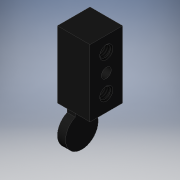
# Autodesk Inventor part: HGP-16---(116_JAW)
Saved by Autodesk Inventor 2019 (Build 230136000, 136)
## iProperties
Created: 2023-03-06
Part Number: HGP-16---(116_JAW)
Material: Generic
Catalog Web Link: www.cadenas.de
Description: HGP-(JAW)-parallel gripper
Vendor: FESTO
Document SubType Name: Modeling
Designer: psAdmin
Manufacturer: FESTO
Mass: 2.0446 g
Surface Area: 15.2758 cm^2
Volume: 2.0446 cm^3
Density: 1 g/cm^3
Appearance: PSOLRGB-128-128-128
Category: PARTsolutions
Company: FESTO
Title: HGP-16
Author: Cadenas PARTsolutions
Comments: parallel gripper
PSOL_IDENT_0: {$CADENAS_DATA/23d-libs/festo/parts/h/hgp/parts/hgp_jaw.prj},168 {VTYP=3D},{NB=HGP-16---(116_JAW)},{
PSOL_IDENT_1: LINA=HGP-16},{NN=HGP-(JAW)},{DATE=10.09.2021 08:18:21},{GEOMDATE=11.03.2020 13:19:07},{VERSION=},{LI
PSOL_IDENT_2: NEID=210},{WBVAR=},{WBNUMERIC=}  {NB=HGP-16---(116_JAW)},{LINA=HGP-16},{KT=3},{TNR=},{TYP=HGP-16},{K
PSOL_IDENT_3: DM=116},{B1=47.000},{B2=25.000},{B3=16.400},{B4=43.800},{B5=46.400},{B6=10.000},{B8=67.000},{D2=M 4}
PSOL_IDENT_4: ,{D4=M 4},{D5=3.300},{D6=3.000},{H1=83.000},{H2=20.500},{H7=11.000},{H8=5.500},{H9=10.000},{H11=38.1
PSOL_IDENT_5: 00},{L3=10.000},{L6S=30.000},{D4P=4.000},{KDR5=3.242},{VERS=3.000}
NB: HGP-16---(116_JAW)
NN: HGP-(JAW)
NT: parallel gripper
NBSYN: $TYP.---($KDM._JAW)
LINA: HGP-16
CATALOG: Festo
TYP: HGP-16
KDM: 116
B1: 47
B2: 25
B3: 16.4
B4: 43.8
B5: 46.4
B6: 10
B8: 67
D2: M 4
D4: M 4
D5: 3.3
D6: 3
H1: 83
H2: 20.5
H7: 11
H8: 5.5
H9: 10
H11: 38.1
L3: 10
L6S: 30
D4P: 4
SUPPLIER: FESTO
ARTICLENO: HGP-16---(116_JAW)
BOMINFO: HGP-16
CREATOR: CADENAS GmbH
Autodesk Inventor part; units mm, degrees
sketch "Sketch_11" plane through (0, 0, 0) normal (0, 0, 1) x (1, 0, 0)
  line L0 (0, 0) -> (10, 0)
  line L1 (10, 0) -> (10, 20.5)
  line L2 (10, 20.5) -> (0, 20.5)
  line L3 (0, 20.5) -> (0, 0)
  constraints: 8 end point
extrude "Extrusion1" add sketch "Sketch_11" along normal mid plane 10
sketch "Sketch2" plane through (0, 0, 5) normal (-1, 0, 0) x (0, 0, 1)
  point P0 (-5, 10.5)
hole "Hole1" at (0, 10.5, 0) direction (1, 0, 0) diameter 3 depth 10
sketch "Sketch_16" plane through (0, 0, 0) normal (0, 0, 1) x (1, 0, 0)
  line L0 (10, 5) -> (0, 5)
  line L1 (0, 5) -> (0, 7)
  line L2 (0, 7) -> (0.379, 6.621)
  line L3 (0.379, 6.621) -> (9.621, 6.621)
  line L4 (9.621, 6.621) -> (10, 7)
  line L5 (10, 7) -> (10, 5)
  line L6 (10, 5) -> (0, 5)
  constraints: 14 end point
revolve "Revolution1" cut sketch "Sketch_16" angle 360 about axis through (10, 5, 0) along (-1, 0, 0)
thread "Thread1" size "M4x0.7" class "6H" standard "ISO Metric profile" full length
sketch "Sketch_17" plane through (0, 0, 0) normal (0, 0, 1) x (1, 0, 0)
  line L0 (10, 16) -> (0, 16)
  line L1 (0, 16) -> (0, 18)
  line L2 (0, 18) -> (0.379, 17.621)
  line L3 (0.379, 17.621) -> (9.621, 17.621)
  line L4 (9.621, 17.621) -> (10, 18)
  line L5 (10, 18) -> (10, 16)
  line L6 (10, 16) -> (0, 16)
  constraints: 14 end point
revolve "Revolution2" cut sketch "Sketch_17" angle 360 about axis through (10, 16, 0) along (-1, 0, 0)
thread "Thread2" size "M4x0.7" class "6H" standard "ISO Metric profile" full length
sketch "Sketch_1" plane through (0, 0, 0) normal (1, 0, 0) x (0, 1, 0)
  arc A0 (-4, 2) -> (-4, -2) centre (-8.5826, 0) ccw
  line L0 (-4, -2) -> (0, -2)
  line L1 (0, -2) -> (0, 2)
  line L2 (0, 2) -> (-4, 2)
  constraints: 6 end point, 2 point on circle, 1 centre point
extrude "Extrusion2" add sketch "Sketch_1" along normal blind 2.5
ref_plane "ANBAU_XY" through (0, 0, 0) normal (-1, 0, 0) x (0, 0, -1)
ref_plane "ANBAU_YZ" through (0, 0, 0) normal (0, 0, -1) x (0, -1, 0)
ref_plane "ANBAU_ZX" through (0, 0, 0) normal (0, -1, 0) x (-1, 0, 0)
body "Solid1"
